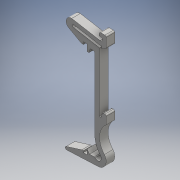
# Autodesk Inventor part: raspDinClipmmv2
Saved by Autodesk Inventor 2016 (Build 200138000, 138)
## iProperties
Created: 2016-08-27
Part Number: raspDinClipmmv2
Material: Generic
Document SubType Name: Modeling
Designer: Thetheos
Density: 1 g/cm^3
Appearance: Default
Author: Thetheos
Autodesk Inventor part; units mm, degrees
ref_plane "YZ Plane" through (0, 0, 0) normal (1, 0, 0) x (0, 1, 0)
ref_plane "XZ Plane" through (0, 0, 0) normal (0, 1, 0) x (-1, 0, 0)
ref_plane "XY Plane" through (0, 0, 0) normal (0, 0, 1) x (1, 0, 0)
sketch "Sketch1" plane through (0, 0, 0) normal (0, 1, 0) x (-1, 0, 0)
  arc A0 (-159.7794, 702.6597) -> (-160.5669, 701.8721) centre (-159.7794, 701.8721) ccw
  line L0 (-155.7462, 702.6597) -> (-155.7462, 704.2667)
  line L1 (-155.7462, 704.2667) -> (-153.4941, 704.2667)
  line L2 (-153.4941, 704.2667) -> (-153.4941, 702.7805)
  line L3 (-153.4941, 702.7805) -> (-152.5972, 702.7805)
  arc A1 (-164.1836, 648.4268) -> (-160.5669, 657.8731) centre (-174.7114, 657.8731) ccw
  line L4 (-160.5669, 657.8731) -> (-160.5669, 701.8721)
  arc A2 (-160.1794, 645.8656) -> (-160.7583, 645.6139) centre (-160.1783, 645.0714) ccw
  arc A3 (-164.1836, 648.4268) -> (-160.7583, 645.6139) centre (-162.4137, 647.0901) ccw
  line L5 (-155.7462, 645.8656) -> (-155.7462, 644.7447)
  line L6 (-155.7462, 644.7447) -> (-153.4959, 644.7447)
  line L7 (-153.4959, 644.7447) -> (-153.4959, 645.7914)
  arc A4 (-143.0499, 641.0266) -> (-142.8493, 642.7649) centre (-143.1468, 641.9185) ccw
  line L8 (-163.0475, 641.9081) -> (-143.0499, 641.0266)
  arc A5 (-166.5264, 650.2868) -> (-163.0475, 641.9081) centre (-162.4021, 647.0877) ccw
  arc A6 (-166.5264, 650.2868) -> (-167.6429, 666.7468) centre (-174.8334, 657.9912) ccw
  line L9 (-167.6429, 666.7468) -> (-167.6429, 671.3153)
  arc A7 (-166.8471, 672.1213) -> (-167.6429, 671.3153) centre (-166.8257, 671.3043) ccw
  line L10 (-166.8471, 672.1213) -> (-166.0512, 672.1176)
  arc A8 (-165.304, 671.5825) -> (-166.0512, 672.1176) centre (-166.0579, 671.319) ccw
  line L11 (-165.304, 671.5825) -> (-164.5204, 669.4361)
  line L12 (-164.5204, 669.4361) -> (-164.4882, 669.3468)
  arc A9 (-164.4882, 669.3468) -> (-164.2374, 669.1723) centre (-164.2343, 669.4443) ccw
  line L13 (-164.2374, 669.1723) -> (-163.8302, 669.1723)
  arc A10 (-163.8326, 669.1723) -> (-163.5671, 669.4384) centre (-163.8364, 669.4416) ccw
  line L14 (-163.5671, 669.4384) -> (-163.5671, 706.0242)
  line L15 (-163.5671, 706.0242) -> (-163.5671, 706.0613)
  line L16 (-163.5671, 706.0613) -> (-147.5434, 708.8923)
  arc A11 (-147.5434, 708.8923) -> (-147.8025, 710.4755) centre (-147.5845, 709.6983) ccw
  line L17 (-147.8025, 710.4755) -> (-163.5671, 707.6952)
  line L18 (-163.5671, 707.6952) -> (-164.9603, 707.6952)
  line L19 (-164.9603, 707.6952) -> (-164.9605, 706.5472)
  arc A12 (-165.374, 706.3282) -> (-164.9605, 706.5472) centre (-165.23, 706.5562) ccw
  line L20 (-165.374, 706.3282) -> (-167.226, 707.3966)
  arc A13 (-167.6397, 708.1008) -> (-167.226, 707.3966) centre (-166.8384, 708.0979) ccw
  line L21 (-167.6397, 708.1008) -> (-167.6393, 713.6964)
  arc A14 (-166.8357, 714.5011) -> (-167.6393, 713.6964) centre (-166.8345, 713.6963) ccw
  line L22 (-166.8357, 714.5011) -> (-164.1567, 714.5011)
  arc A15 (-163.353, 713.6974) -> (-164.1567, 714.5011) centre (-164.1583, 713.6958) ccw
  line L23 (-163.353, 713.6974) -> (-163.353, 712.3579)
  line L24 (-163.353, 712.3579) -> (-165.4962, 711.98)
  line L25 (-165.4962, 711.98) -> (-165.4962, 711.7118)
  arc A16 (-165.4962, 711.7118) -> (-163.8213, 710.1096) centre (-163.8924, 711.7118) ccw
  line L26 (-163.8213, 710.1096) -> (-146.2918, 713.1784)
  arc A17 (-144.5878, 707.1017) -> (-146.2918, 713.1784) centre (-146.018, 709.9779) ccw
  arc A18 (-152.5972, 702.7805) -> (-152.2275, 702.8725) centre (-152.6033, 703.5935) ccw
  line L27 (-155.7462, 702.6597) -> (-155.7462, 700.1597)
  line L28 (-155.7462, 700.1597) -> (-156.9462, 700.1597)
  line L29 (-156.9462, 700.1597) -> (-157.7628, 702.6597)
  line L30 (-157.7628, 702.6597) -> (-159.7794, 702.6597)
  line L31 (-155.7462, 645.8656) -> (-155.7462, 647.8656)
  line L32 (-155.7462, 647.8656) -> (-157.3545, 645.8656)
  line L33 (-157.3545, 645.8656) -> (-160.1794, 645.8656)
  line L34 (-142.8493, 642.7649) -> (-152.5613, 645.7914)
  line L35 (-144.5878, 707.1017) -> (-152.2275, 702.8725)
  line L36 (-152.5613, 645.7914) -> (-153.4959, 645.7914)
  point P0 (-160.5669, 683.588)
  dimension "d2" = 43.999
  dimension "d3" = 3.0002
  dimension "d6" = 2.5
  dimension "d7" = 1.2
  dimension "d8" = 2
  constraints: 74 end point, 39 point on circle, 19 centre point, 6 perpendicular, 3 horizontal, 3 vertical, 1 point on line, 1 tangent
  measures "d2" distance of L4.start L4.end
  measures "d3" distance between parallel lines of L14 L4
  measures "d6" distance of L0.start L27.end
  measures "d7" distance of L27.end L28.end
  measures "d8" distance of L5.start L31.end
extrude "Extrusion1" add sketch "Sketch1" along normal blind 5.3
body "Solid1"
